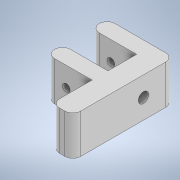
# Autodesk Inventor part: Idle belt holder
Saved by Autodesk Inventor 2022 (Build 260153000, 153)
## iProperties
Created: 2021-10-05
Part Number: Idle belt holder
Material: Generic
Document SubType Name: Modeling
Designer: Administrator
Density: 1 g/cm^3
Appearance: Default
Mass: 4.75917 g
Surface Area: 26.3693 cm^2
Volume: 4.75917 cm^3
Title: Idle belt holder v4
Author: Administrator
Autodesk Inventor part; units mm, degrees
ref_plane "YZ Plane" through (0, 0, 0) normal (1, 0, 0) x (0, 1, 0)
ref_plane "XY Plane" through (0, 0, 0) normal (0, 0, 1) x (1, 0, 0)
ref_plane "Work Plane1" through (0, -6.5, 0) normal (0, 1, 0) x (-1, 0, 0)
sketch "Sketch1" plane through (0, -6.5, 0) normal (0, 1, 0) x (-1, 0, 0)
  arc A0 (-22, -3.125) -> (-19.375, -5.75) centre (-19.375, -3.125) ccw
  line L0 (-22, -3.125) -> (-22, 24.975)
  arc A1 (-19.375, 27.6) -> (-22, 24.975) centre (-19.375, 24.975) ccw
  line L1 (-15, 24.975) -> (-15, 14.25)
  line L2 (-2.625, 9) -> (-15, 9)
  line L3 (-19.375, 27.6) -> (-17.625, 27.6)
  line L4 (-15, 9) -> (-15, -0.5)
  arc A2 (-15, 24.975) -> (-17.625, 27.6) centre (-17.625, 24.975) ccw
  line L5 (-15, 14.25) -> (-2.625, 14.25)
  line L6 (-2.625, -5.75) -> (-19.375, -5.75)
  arc A3 (-2.625, 9) -> (-2.625, 14.25) centre (-2.625, 11.625) ccw
  line L7 (-15, -0.5) -> (-2.625, -0.5)
  arc A4 (-2.625, -5.75) -> (-2.625, -0.5) centre (-2.625, -3.125) ccw
  constraints: 16 end point, 10 point on circle, 5 centre point, 5 horizontal, 4 equal radius, 3 vertical, 2 parallel, 1 collinear
extrude "Extrusion2" add sketch "Sketch1" along normal blind 13
sketch "Sketch2" plane through (15, -6.5, 14.25) normal (-1, 0, 0) x (0, 0, 1)
  circle A0 centre (-10, 6.5) radius 3.25
  constraints: 1 centre point
extrude "Extrusion1" cut sketch "Sketch2" against normal blind 3
hole "Hole3" at (6.5, 0, 9) direction (0, 0, 1) diameter 2.529 depth 5.25 tip angle 118
sketch "Sketch4" plane through (22, -6.5, 24.975) normal (1, 0, 0) x (0, 0, -1)
  point P0 (20.725, 6.5)
hole "Hole2" at (22, 0, 4.25) direction (-1, 0, 0) diameter 3.4 depth 4 tip angle 118
sketch "Sketch3" plane through (15, -6.5, 9) normal (0, 0, -1) x (-1, 0, 0)
  point P0 (8.5, 6.5)
hole "Hole1" at (6.5, 0, -5.75) direction (0, 0, 1) diameter 2.529 depth 5.25 tip angle 118
sketch "Sketch5" plane through (19.375, -6.5, -5.75) normal (0, 0, -1) x (-1, 0, 0)
  point P0 (12.875, 6.5)
body "Solid3"
